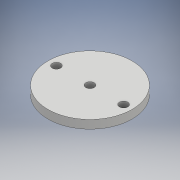
# Autodesk Inventor part: кривошип_v2
Saved by Autodesk Inventor 2017.3 (Build 213256000, 256)
## iProperties
Part Number: кривошип_v2
Material: Типовые
Document SubType Name: Modeling
Designer: Alexnav
Density: 1 g/cm^3
Appearance: По умолчанию
Mass: 76.1836 g
Surface Area: 193.208 cm^2
Volume: 76.1836 cm^3
Author: Alexnav
Autodesk Inventor part; units mm, degrees
ref_plane "YZ Plane" through (0, 0, 0) normal (1, 0, 0) x (0, 1, 0)
ref_plane "XZ Plane" through (0, 0, 0) normal (0, 1, 0) x (-1, 0, 0)
ref_plane "XY Plane" through (0, 0, 0) normal (0, 0, 1) x (1, 0, 0)
sketch "Эскиз1" plane through (0, 0, 0) normal (0, 0, 1) x (1, 0, 0)
  circle A0 centre (0, 0) radius 50
  dimension "d0" = 100
  constraints: 1 centre point, 1 coincident
  measures "d0" diameter of A0
extrude "Выдавливание1" add sketch "Эскиз1" along normal blind 10
sketch "Эскиз3" plane through (0, 0, 10) normal (0, 0, 1) x (1, 0, 0)
  line L0 (-70, 0) -> (70, 0) projected
  circle A0 centre (0, 0) radius 5
  circle A1 centre (-40, 0) radius 5
  circle A2 centre (40, 0) radius 5
  line L1 (0, -70) -> (0, 70) projected
  dimension "d7" = 40
  dimension "d8" = 10
  constraints: 3 centre point, 2 equal radius, 2 point on line, 1 coincident, 1 symmetric about line
  measures "d7" distance of A1.centre point (0, 0)
  measures "d8" diameter of A0
extrude "Выдавливание3" cut sketch "Эскиз3" against normal through all
